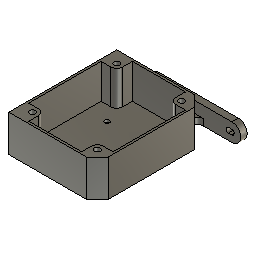
card-reader-mount (Autodesk Fusion 360 design; units mm, degrees)
Autodesk Fusion 360 part; units mm, degrees
sketch "Sketch1" plane through (0, 0, 0) normal (0, 0, 1) x (1, 0, 0)
  line L0 (-41, 50) -> (-41, -50)
  line L1 (-41, -50) -> (31, -50)
  line L2 (31, -50) -> (41, -40)
  line L3 (41, -40) -> (41, 40)
  line L4 (41, 40) -> (31, 50)
  line L5 (31, 50) -> (-41, 50)
  line L6 (-30, 39) -> (30, 39) construction
  line L7 (30, 39) -> (30, -39) construction
  line L8 (30, -39) -> (-30, -39) construction
  line L9 (-30, -39) -> (-30, 39) construction
  line L10 (0, -39) -> (0, 39) construction
  line L11 (-41, 0) -> (41, 0) construction
  circle A0 centre (-30, 39) radius 2.665
  circle A1 centre (30, 39) radius 2.665
  circle A2 centre (30, -39) radius 2.665
  circle A3 centre (-30, -39) radius 2.665
  line L12 (30.1716, -48) -> (39, -39.1716)
  line L13 (39, -39.1716) -> (39, 39.1716)
  line L14 (39, 39.1716) -> (30.1716, 48)
  line L15 (30.1716, 48) -> (-39, 48)
  line L16 (-39, 48) -> (-39, -48)
  line L17 (-39, -48) -> (30.1716, -48)
  line L18 (-14, 37) -> (14, 37) construction
  line L19 (29, 22) -> (29, -22) construction
  line L20 (14, -37) -> (-14, -37) construction
  line L21 (-29, -22) -> (-29, 22) construction
  line L22 (-29, 0) -> (29, 0) construction
  arc A4 (29, 22) -> (14, 37) centre (14, 22) ccw construction
  arc A5 (-14, 37) -> (-29, 22) centre (-14, 22) ccw construction
  arc A6 (-29, -22) -> (-14, -37) centre (-14, -22) ccw construction
  arc A7 (14, -37) -> (29, -22) centre (14, -22) ccw construction
  arc A8 (24.5, 39) -> (30, 33.5) centre (30, 39) ccw
  arc A9 (30, -33.5) -> (24.5, -39) centre (30, -39) ccw
  line L23 (24.5, -48) -> (24.5, -39)
  line L24 (39, -33.5) -> (30, -33.5)
  line L25 (39, 33.5) -> (30, 33.5)
  line L26 (24.5, 39) -> (24.5, 48)
  arc A10 (-24.5, -39) -> (-30, -33.5) centre (-30, -39) ccw
  arc A11 (-30, 33.5) -> (-24.5, 39) centre (-30, 39) ccw
  line L27 (-30, 33.5) -> (-39, 33.5)
  line L28 (-24.5, 39) -> (-24.5, 48)
  line L29 (-30, -33.5) -> (-39, -33.5)
  line L30 (-24.5, -39) -> (-24.5, -48)
  line L31 (-15, -48) -> (15, -48)
  line L32 (15, -48) -> (15, -33)
  line L33 (15, -33) -> (-15, -33)
  line L34 (-15, -33) -> (-15, -48)
  point P0 (-29, 37)
  point P1 (29, 37)
  point P2 (-29, -37)
  point P3 (0, -33)
  dimension "d1" = 60
  dimension "d2" = 78
  dimension "d3" = 82
  dimension "d4" = 100
  dimension "d5" = 135
  dimension "d6" = 10
  dimension "d8" = 5.33
  dimension "d10" = 58
  dimension "d11" = 74
  dimension "d12" = 15
  dimension "d19" = 5.5
  dimension "d53" = 30
  dimension "d54" = 15
  constraint vertical L0
  constraint horizontal L1
  constraint vertical L3
  constraint horizontal L5
  constraint horizontal L6
  constraint vertical L7
  constraint horizontal L8
  constraint vertical L9
  constraint midpoint L8 L10.start
  constraint midpoint L6 L10.end
  constraint midpoint L0 L11.start
  constraint midpoint L3 L11.end
  constraint midpoint L10 L11
  constraint symmetric L2 L4 L11
  constraint midpoint origin L11
  constraint coincident L6.start L9.end
  constraint coincident L6.end L7.start
  constraint coincident L7.end L8.start
  constraint coincident L8.end L9.start
  constraint equal A0 A1
  constraint equal A2 A3
  constraint equal A0 A3
  constraint horizontal L18
  constraint vertical L19
  constraint horizontal L20
  constraint vertical L21
  constraint coincident P1 L18
  constraint coincident P1 L19
  constraint tangent L18 A4
  constraint tangent L19 A4
  constraint coincident L21 L22.start
  constraint coincident P0 L18
  constraint coincident P0 L21
  constraint tangent L18 A5
  constraint tangent L21 A5
  constraint equal A4 A5
  constraint coincident P2 L20
  constraint coincident P2 L21
  constraint tangent L20 A6
  constraint tangent L21 A6
  constraint equal A4 A6
  constraint tangent L19 A7
  constraint tangent L20 A7
  constraint equal A4 A7
  constraint midpoint L19 L22.end
  constraint midpoint L21 L22.start
  constraint midpoint origin L22
  constraint coincident L17 L23.start
  constraint coincident L13 L24.start
  constraint coincident A9.start L24.end
  constraint coincident A9.end L23.end
  constraint tangent A9 L23
  constraint tangent A9 L24
  constraint horizontal L24
  constraint vertical L23
  constraint coincident L13 L25.start
  constraint coincident L15 L26.end
  constraint horizontal L25
  constraint vertical L26
  constraint tangent A8 L26
  constraint tangent A8 L25
  constraint coincident L16 L27.end
  constraint coincident L15 L28.end
  constraint coincident L16 L29.end
  constraint vertical L28
  constraint horizontal L27
  constraint horizontal L29
  constraint vertical L30
  constraint coincident L17 L30.end
  constraint tangent A10 L30
  constraint tangent A10 L29
  constraint tangent A11 L27
  constraint tangent A11 L28
  constraint equal A9 A10
  constraint equal A8 A11
  constraint equal A10 A11
  constraint horizontal L31
  constraint vertical L32
  constraint horizontal L33
  constraint vertical L34
  constraint midpoint L33 P3
  constraint coincident L12.start L31
  constraint coincident L10 P3
  measures "d1" distance of L6.start L6.end
  measures "d2" distance of L6.end L7.end
  measures "d3" distance of L0 L3
  measures "d4" distance of L0.start L0.end
  measures "d5" angle of L4 L5
  measures "d6" distance of L3.end L5
  measures "d8" diameter of A0
  measures "d10" distance of P0 P1
  measures "d11" distance of P0 P2
  measures "d12" radius of A4
  measures "d19" radius of A11
  measures "d53" distance of L32.end L33.end
  measures "d54" distance of L31.start L33.end
extrude "Extrude1" add sketch "Sketch1" along normal blind 2 contours L0 L1 L2 L3 L4 L5 | A0 | A1 | A2 | A3 | L12 L13 L17 A9 L23 L24 | L13 L15 L16 L17 A8 A9 L23 L24 L25 L26 A10 A11 L27 L28 L29 L30 L32 L33 L34 | L13 L14 L15 A8 L25 L26 | L16 L17 A10 L29 L30 | L15 L16 A11 L27 L28 makes body 1
extrude "Extrude2" add sketch "Sketch1" along normal blind 34 contours L0 L1 L2 L3 L4 L5 | A0 | A1 | A2 | A3 | L12 L13 L17 A9 L23 L24 | L13 L14 L15 A8 L25 L26 | L16 L17 A10 L29 L30 | L15 L16 A11 L27 L28 bodies 1
extrude "Extrude3" cut sketch "Sketch1" against normal blind 15 from surface at 34 contours A0 | A1 | A2 | A3 bodies 1
fillet "Fillet2" radius 4 2 edges at (-15, -33, 1) (15, -33, 1) on bodies 1
sketch "Sketch3" plane through (0, 0, 0) normal (0, 0, 1) x (1, 0, 0)
  line L0 (20, 20) -> (-20, 20) construction
  line L1 (-20, 20) -> (-20, -20) construction
  line L2 (-20, -20) -> (20, -20) construction
  line L3 (20, -20) -> (20, 20) construction
  line L4 (20, 0) -> (-20, 0) construction
  circle A0 centre (20, 20) radius 2.665
  circle A1 centre (-20, 20) radius 2.665
  circle A2 centre (-20, -20) radius 2.665
  circle A3 centre (20, -20) radius 2.665
  arc A4 (28, 20) -> (20, 28) centre (20, 20) ccw
  arc A5 (-20, 28) -> (-28, 20) centre (-20, 20) ccw
  arc A6 (-28, -20) -> (-20, -28) centre (-20, -20) ccw
  arc A7 (20, -28) -> (28, -20) centre (20, -20) ccw
  line L5 (28, -20) -> (28, 20)
  line L6 (20, 28) -> (-20, 28)
  line L7 (-28, 20) -> (-28, -20)
  line L8 (-20, -28) -> (20, -28)
  line L9 (31, 50) -> (-41, 50) construction
  line L10 (15, 75) -> (-15, 75)
  line L11 (-15, 75) -> (-15, 28)
  line L12 (-15, 28) -> (15, 28)
  line L13 (15, 28) -> (15, 75)
  line L14 (15, 50) -> (-15, 50) construction
  line L15 (0, 50) -> (0, 75) construction
  line L16 (7, 61.5) -> (7, 57.5) construction
  arc A8 (8.5, 61.5) -> (5.5, 61.5) centre (7, 61.5) ccw
  arc A9 (5.5, 57.5) -> (8.5, 57.5) centre (7, 57.5) ccw
  line L17 (8.5, 57.5) -> (8.5, 61.5)
  line L18 (5.5, 61.5) -> (5.5, 57.5)
  line L19 (-8.5, 57.5) -> (-8.5, 61.5)
  arc A10 (-5.5, 61.5) -> (-8.5, 61.5) centre (-7, 61.5) ccw
  arc A11 (-8.5, 57.5) -> (-5.5, 57.5) centre (-7, 57.5) ccw
  line L20 (-5.5, 61.5) -> (-5.5, 57.5)
  line L21 (7, 57.5) -> (15, 57.5) construction
  arc A12 (15, 33) -> (20, 28) centre (20, 33) ccw
  arc A13 (-20, 28) -> (-15, 33) centre (-20, 33) ccw
  line L22 (-15, 69) -> (15, 69) construction
  line L23 (7, 69) -> (7, 61.5) construction
  line L24 (7, 50) -> (7, 57.5) construction
  point P0 (7, 59.5)
  dimension "d24" = 40
  dimension "d25" = 40
  dimension "d26" = 5.33
  dimension "d28" = 8
  dimension "d32" = 30
  dimension "d48" = 25
  dimension "d50" = 1.5
  dimension "d51" = 4
  dimension "d66" = 7
  dimension "d67" = 6
  constraint horizontal L0
  constraint vertical L1
  constraint horizontal L2
  constraint vertical L3
  constraint midpoint L3 L4.start
  constraint midpoint L1 L4.end
  constraint midpoint origin L4
  constraint coincident L0.start L3.end
  constraint coincident L0.end L1.start
  constraint coincident L1.end L2.start
  constraint coincident L2.end L3.start
  constraint equal A0 A1
  constraint equal A0 A3
  constraint equal A2 A3
  constraint equal A4 A5
  constraint equal A6 A7
  constraint equal A4 A7
  constraint tangent A5 L6
  constraint tangent A4 L6
  constraint tangent A6 L8
  constraint tangent A7 L8
  constraint tangent A4 L5
  constraint tangent A7 L5
  constraint tangent A5 L7
  constraint tangent A6 L7
  constraint horizontal L10
  constraint vertical L11
  constraint horizontal L12
  constraint vertical L13
  constraint midpoint L6 L12
  constraint coincident L13 L14.start
  constraint coincident L11 L14.end
  constraint horizontal L14
  constraint coincident L9.end L14
  constraint midpoint L14 L15.start
  constraint midpoint L10 L15.end
  constraint coincident L16.start A8.centre
  constraint coincident L16.end A9.centre
  constraint equal A8 A9
  constraint vertical L16
  constraint midpoint L16 P0
  constraint vertical L18
  constraint vertical L17
  constraint tangent A8 L17
  constraint tangent A8 L18
  constraint symmetric L15 A8.start L19.end
  constraint symmetric L15 A8.end A10.start
  constraint symmetric L15 A8 A10
  constraint symmetric L15 A9.start A11.end
  constraint symmetric L15 A9.end L19.start
  constraint symmetric L15 A9 A11
  constraint coincident L13 L21.end
  constraint horizontal L21
  constraint coincident A4.end L6.start
  constraint coincident L13 A12.start
  constraint tangent A4 A12
  constraint tangent L13 A12
  constraint coincident A5.start L6.end
  constraint coincident L11 A13.end
  constraint tangent A5 A13
  constraint tangent L11 A13
  constraint coincident L11 L22.start
  constraint coincident L13 L22.end
  constraint horizontal L22
  constraint coincident L22 L23.start
  constraint coincident L14 L24.start
  constraint vertical L23
  constraint vertical L24
  constraint equal L23 L24
  measures "d24" distance of L0.start L0.end
  measures "d25" distance of L0.start L2.end
  measures "d26" diameter of A0
  measures "d28" radius of A4
  measures "d32" distance of L10.start L10.end
  measures "d48" distance of L10 L14
  measures "d50" radius of A8
  measures "d51" distance of L16.start L16.end
  measures "d66" distance of L15 L16
  measures "d67" distance of L10 L22
sketch "Sketch7" plane through (0, 0, 0) normal (0, 0, 1) x (1, 0, 0)
  circle A0 centre (-20, 20) radius 2.25
  circle A1 centre (20, 20) radius 2.25
  circle A2 centre (20, -20) radius 2.25
  circle A3 centre (-20, -20) radius 2.25
  point P0 (-20, 20)
  point P1 (20, 20)
  point P2 (20, -20)
  point P3 (-20, -20)
  dimension "d61" = 4.5
  constraint coincident P0 A0.centre
  constraint coincident P1 A1.centre
  constraint coincident P2 A2.centre
  constraint coincident P3 A3.centre
  constraint equal A0 A1
  constraint equal A2 A3
  constraint equal A0 A3
  measures "d61" diameter of A0
extrude "Extrude7" cut sketch "Sketch7" along normal through all bodies 1
copy_body "Body->Comp1" bodies 1 removing the originals makes body 2 in component "Box"
extrude "Extrude5" add sketch "Sketch3" against normal blind 6 separate body makes body 3
sketch "Sketch4" plane through (0, 75, 0) normal (0, 1, 0) x (-1, 0, 0)
  line L0 (15, 0) -> (-15, 0)
  line L1 (15, -6) -> (15, 0)
  line L2 (-15, -6) -> (15, -6)
  line L3 (-15, 0) -> (-15, -6)
  arc A0 (26.5, -6) -> (26.5, 10.5) centre (26.5, 2.25) ccw
  arc A1 (-46.5, 10.5) -> (-46.5, -6) centre (-46.5, 2.25) ccw
  line L4 (26.5, 10.5) -> (-46.5, 10.5)
  line L5 (-46.5, -6) -> (26.5, -6)
  line L6 (26.5, 4.5) -> (23.5, 4.5)
  line L7 (23.5, 0) -> (26.5, 0)
  line L8 (26.5, 2.25) -> (23.5, 2.25) construction
  arc A2 (26.5, 0) -> (26.5, 4.5) centre (26.5, 2.25) ccw
  arc A3 (23.5, 4.5) -> (23.5, 0) centre (23.5, 2.25) ccw
  line L9 (-10, 10.5) -> (-10, -6) construction
  arc A4 (-43.5, 0) -> (-43.5, 4.5) centre (-43.5, 2.25) ccw
  arc A5 (-46.5, 4.5) -> (-46.5, 0) centre (-46.5, 2.25) ccw
  line L10 (-43.5, 0) -> (-46.5, 0)
  line L11 (-46.5, 4.5) -> (-43.5, 4.5)
  point P0 (25, 2.25)
  point P1 (-45, 2.25)
  point P2 (0, -6)
  dimension "d39" = 4.5
  dimension "d40" = 6
  dimension "d41" = 3
  dimension "d43" = 70
  dimension "d57" = 10
  constraint horizontal L5
  constraint horizontal L4
  constraint tangent A0 L5
  constraint tangent A0 L4
  constraint tangent A1 L4
  constraint tangent A1 L5
  constraint horizontal L6
  constraint horizontal L7
  constraint horizontal L8
  constraint coincident A0.centre L8.start
  constraint coincident L8.end A3.centre
  constraint coincident L6 A2.end
  constraint coincident L6.end A3.start
  constraint coincident L6.start A2.end
  constraint midpoint L4 L9.start
  constraint equal A2 A3
  constraint tangent L7 A2
  constraint tangent L6 A3
  constraint midpoint L8 P0
  constraint symmetric L6.start L9 A5.start
  constraint symmetric L6.end L9 A4.end
  constraint symmetric L7.start L9 A4.start
  constraint symmetric L7.end L9 A5.end
  constraint symmetric A2 L9 A5
  constraint symmetric A3 L9 A4
  constraint symmetric L9 P0 P1
  constraint midpoint L5 L9.end
  constraint collinear L2 L5
  constraint midpoint L2 P2
  measures "d39" distance of L6 L7
  measures "d40" distance of A0 A2
  measures "d41" distance of A0.centre L8.end
  measures "d43" distance of P0 P1
  measures "d57" distance of L9 P2
extrude "Extrude6" add sketch "Sketch4" against normal blind 6 bodies 3
fillet "Fillet3" radius 5 2 edges at (-15, 69, -3) (15, 69, -3) on bodies 3
copy_body "Body->Comp2" bodies 3 removing the originals makes body 4 in component "Mount"
component "Box" placed x (1, 0, 0) y (0, 1, 0) z (0, 0, 1) at (0, 0, 0)
component "Mount" placed x (1, 0, 0) y (0, 1, 0) z (0, 0, 1) at (0, 0, 0)
equation "d5 = 180 deg - 45 deg"
equation "BoxWallThickness = 2 mm"
equation "d8 = InsertDiameter"
equation "d9 = -BoxWallThickness"
equation "BoxDepth = 34 mm"
equation "d15 = BoxWallThickness"
equation "d17 = BoxDepth"
equation "d26 = InsertDiameter"
equation "MountThickness = 6 mm"
equation "d36 = -MountThickness"
equation "d40 = MountThickness"
equation "d44 = -MountThickness"
equation "d50 = ( 3 / 2 ) * 1 mm"
equation "InsertDiameter = 5.33 mm"
equation "InsertDepth = 6.5 mm"
equation "d67 = MountThickness"
